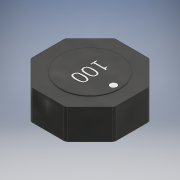
# Autodesk Inventor part: 34-103B
Saved by Autodesk Inventor 2018 (Build 220112000, 112)
## iProperties
Created: 2019-11-06
Part Number: 34-103B
Material: Iron, Cast
Document SubType Name: Modeling
Designer: Bradley
Density: 7.15 g/cm^3
Appearance: Fine Textured - Black
Author: Bradley
Autodesk Inventor part; units mm, degrees
ref_plane "YZ Plane" through (0, 0, 0) normal (1, 0, 0) x (0, 1, 0)
ref_plane "XZ Plane" through (0, 0, 0) normal (0, 1, 0) x (-1, 0, 0)
ref_plane "XY Plane" through (0, 0, 0) normal (0, 0, 1) x (1, 0, 0)
sketch "Sketch1" plane through (0, 0, 0) normal (0, 0, 1) x (1, 0, 0)
  circle A0 centre (0, 0) radius 3.5
  dimension "d0" = 7
  constraints: 1 centre point, 1 coincident
  measures "d0" diameter of A0
extrude "Extrusion1" add sketch "Sketch1" along normal mid plane 3.8
sketch "Sketch2" plane through (0, 0, 0) normal (0, 0, 1) x (1, 0, 0)
  line L0 (2.0711, 5) -> (5, 2.0711)
  line L1 (5, 2.0711) -> (5, -2.0711)
  line L2 (5, -2.0711) -> (2.0711, -5)
  line L3 (2.0711, -5) -> (-2.0711, -5)
  line L4 (-2.0711, -5) -> (-5, -2.0711)
  line L5 (-5, -2.0711) -> (-5, 2.0711)
  line L6 (-5, 2.0711) -> (-2.0711, 5)
  line L7 (-2.0711, 5) -> (2.0711, 5)
  point P0 (0, 0)
  point P1 (0, 0)
  dimension "d3" = 10
  constraints: 16 end point, 1 coincident, 1 vertical, 17 other
  measures "d3" distance between parallel lines of L5 L1
extrude "Extrusion2" add sketch "Sketch2" along normal mid plane 3.6
sketch "Sketch3" plane through (0, 0, -1.8) normal (0, 0, -1) x (-1, 0, 0)
  line L0 (-2.0711, 5) -> (-5, 2.0711) projected
  line L1 (-5, 2.0711) -> (-5, -2.0711) projected
  line L2 (-5, -2.0711) -> (-2.0711, -5) projected
  line L3 (-2.0711, -5) -> (2.0711, -5) projected
  line L4 (2.0711, -5) -> (5, -2.0711) projected
  line L5 (5, -2.0711) -> (5, 2.0711) projected
  line L6 (5, 2.0711) -> (2.0711, 5) projected
  line L7 (2.0711, 5) -> (-2.0711, 5) projected
  circle A0 centre (0, 0) radius 3.5 projected
  line L8 (-4.9, -1.6) -> (-3.7, -1.6)
  line L9 (-3.7, -1.6) -> (-3.7, 1.6)
  line L10 (-3.7, 1.6) -> (-4.9, 1.6)
  line L11 (-4.9, 1.6) -> (-4.9, -1.6)
  line L12 (4.9, -1.6) -> (3.7, -1.6)
  line L13 (3.7, -1.6) -> (3.7, 1.6)
  line L14 (3.7, 1.6) -> (4.9, 1.6)
  line L15 (4.9, 1.6) -> (4.9, -1.6)
  point P0 (-4.9, 0)
  point P1 (-5, 0)
  dimension "d6" = 3.2
  dimension "d7" = 0.1
  dimension "d8" = 0.1
  dimension "d9" = 7.4
  constraints: 16 end point, 4 parallel, 2 horizontal, 2 midpoint, 2 perpendicular, 2 point on line, 1 collinear, 1 horizontal alignment
  measures "d6" distance of L10.end L8.start
  measures "d7" distance between parallel lines of L1 L11
  measures "d8" distance between parallel lines of L5 L15
  measures "d9" distance between parallel lines of L13 L9
extrude "Extrusion3" add sketch "Sketch3" along normal blind 0.1 contours L11 L10 L9 L8 | L12 L13 L14 L15
sketch "Sketch4" plane through (0, 0, 1.9) normal (0, 0, 1) x (1, 0, 0)
  circle A0 centre (0, 0) radius 3.5 projected
  circle A1 centre (2.8, 0) radius 0.4
  circle A2 centre (0, 0) radius 3.5 construction
  line L0 (0, 3.5) -> (0, -3.5) construction
  line L1 (-0.8, 0.778) -> (-0.8, 1.5585)
  line L2 (-0.8, 1.5585) -> (-0.6366, 1.5585)
  line L3 (-0.6366, 1.5585) -> (-0.6366, 1.2681)
  line L4 (-0.6366, 1.2681) -> (0.4357, 1.2681)
  line L5 (0.4357, 1.2681) -> (0.4357, 1.5585)
  line L6 (0.4357, 1.5585) -> (0.5822, 1.5585)
  spline S0 degree 2 poles (0.5822, 1.5585) (0.5822, 1.3938) (0.6755, 1.2382) (0.8052, 1.2279) knots 0 0 0 1 2 2 2
  line L7 (0.8052, 1.2279) -> (0.8052, 1.0619)
  line L8 (0.8052, 1.0619) -> (-0.6366, 1.0619)
  line L9 (-0.6366, 1.0619) -> (-0.6366, 0.778)
  line L10 (-0.6366, 0.778) -> (-0.8, 0.778)
  spline S1 degree 2 poles (0, -0.5122) (-0.4305, -0.5122) (-0.8337, -0.2619) (-0.8337, -0.0013) knots 0 0 0 1 2 2 2
  spline S2 degree 2 poles (-0.8337, -0.0013) (-0.8337, 0.2632) (-0.4227, 0.5109) (-0.0013, 0.5109) knots 0 0 0 1 2 2 2
  spline S3 degree 2 poles (-0.0013, 0.5109) (0.4318, 0.5109) (0.8324, 0.2606) (0.8324, -0.0013) knots 0 0 0 1 2 2 2
  spline S4 degree 2 poles (0.8324, -0.0013) (0.8324, -0.2645) (0.4175, -0.5122) (0, -0.5122) knots 0 0 0 1 2 2 2
  spline S5 degree 2 poles (-0.4875, -0.2373) (-0.4084, -0.2684) (-0.1647, -0.2943) (0, -0.2943) knots 0 0 0 1 2 2 2
  spline S6 degree 2 poles (0, -0.2943) (0.1647, -0.2943) (0.4071, -0.2684) (0.4888, -0.236) knots 0 0 0 1 2 2 2
  spline S7 degree 2 poles (0.4888, -0.236) (0.5705, -0.2036) (0.6548, -0.0908) (0.6548, -0.0013) knots 0 0 0 1 2 2 2
  spline S8 degree 2 poles (0.6548, -0.0013) (0.6548, 0.0882) (0.5705, 0.2036) (0.4862, 0.2373) knots 0 0 0 1 2 2 2
  spline S9 degree 2 poles (0.4862, 0.2373) (0.4045, 0.2697) (0.1556, 0.293) (-0.0013, 0.293) knots 0 0 0 1 2 2 2
  spline S10 degree 2 poles (-0.0013, 0.293) (-0.1699, 0.293) (-0.3955, 0.2723) (-0.4836, 0.2386) knots 0 0 0 1 2 2 2
  spline S11 degree 2 poles (-0.4836, 0.2386) (-0.5666, 0.2075) (-0.6561, 0.0921) (-0.6561, -0.0013) knots 0 0 0 1 2 2 2
  spline S12 degree 2 poles (-0.6561, -0.0013) (-0.6561, -0.0895) (-0.5718, -0.2049) (-0.4875, -0.2373) knots 0 0 0 1 2 2 2
  spline S13 degree 2 poles (0, -1.7128) (-0.4305, -1.7128) (-0.8337, -1.4626) (-0.8337, -1.2019) knots 0 0 0 1 2 2 2
  spline S14 degree 2 poles (-0.8337, -1.2019) (-0.8337, -0.9374) (-0.4227, -0.6898) (-0.0013, -0.6898) knots 0 0 0 1 2 2 2
  spline S15 degree 2 poles (-0.0013, -0.6898) (0.4318, -0.6898) (0.8324, -0.94) (0.8324, -1.2019) knots 0 0 0 1 2 2 2
  spline S16 degree 2 poles (0.8324, -1.2019) (0.8324, -1.4652) (0.4175, -1.7128) (0, -1.7128) knots 0 0 0 1 2 2 2
  spline S17 degree 2 poles (-0.4875, -1.4379) (-0.4084, -1.469) (-0.1647, -1.495) (0, -1.495) knots 0 0 0 1 2 2 2
  spline S18 degree 2 poles (0, -1.495) (0.1647, -1.495) (0.4071, -1.469) (0.4888, -1.4366) knots 0 0 0 1 2 2 2
  spline S19 degree 2 poles (0.4888, -1.4366) (0.5705, -1.4042) (0.6548, -1.2914) (0.6548, -1.2019) knots 0 0 0 1 2 2 2
  spline S20 degree 2 poles (0.6548, -1.2019) (0.6548, -1.1125) (0.5705, -0.9971) (0.4862, -0.9634) knots 0 0 0 1 2 2 2
  spline S21 degree 2 poles (0.4862, -0.9634) (0.4045, -0.931) (0.1556, -0.9076) (-0.0013, -0.9076) knots 0 0 0 1 2 2 2
  spline S22 degree 2 poles (-0.0013, -0.9076) (-0.1699, -0.9076) (-0.3955, -0.9284) (-0.4836, -0.9621) knots 0 0 0 1 2 2 2
  spline S23 degree 2 poles (-0.4836, -0.9621) (-0.5666, -0.9932) (-0.6561, -1.1086) (-0.6561, -1.2019) knots 0 0 0 1 2 2 2
  spline S24 degree 2 poles (-0.6561, -1.2019) (-0.6561, -1.2901) (-0.5718, -1.4055) (-0.4875, -1.4379) knots 0 0 0 1 2 2 2
  dimension "d12" = 0.8
  dimension "d13" = 2.8
  constraints: 2 end point, 2 point on circle, 2 vertical, 1 centre point, 1 horizontal alignment, 1 midpoint
  measures "d12" diameter of A1
  measures "d13" distance of A1.centre point (0, 0)
extrude "Extrusion4" add sketch "Sketch4" along normal blind 0.01 contours A1 | L1 L2 L3 L4 L5 L6 S0 L7 L8 L9 L10 | S1 S2 S3 S4 | S13 S14 S15 S16
fillet "Fillet1" radius 0.5 8 edges at (-2.0711, -5, 0) (2.0711, -5, 0) (5, -2.0711, 0) (5, 2.0711, 0) (2.0711, 5, 0) (-2.0711, 5, 0) (-5, 2.0711, 0) (-5, -2.0711, 0)
equation "\"d8\" = d7"
body "Solid1"
